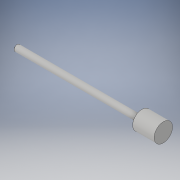
# Autodesk Inventor part: 5.4680.8730.50.500Double acting_00_005.4680.500.75N
Saved by Autodesk Inventor 2019 (Build 230136000, 136)
## iProperties
Created: 2023-02-15
Part Number: 5.4680.8730.50.500Double acting_00_005.4680.500.75N
Material: Generic
Catalog Web Link: www.cadenas.de
Description: SR Series Rod-Pneumatic Cylinder
Vendor: PARKERHANNIFIN
Document SubType Name: Modeling
Designer: psAdmin
Manufacturer: PARKERHANNIFIN
Mass: 10.4158 g
Surface Area: 44.7208 cm^2
Volume: 10.4158 cm^3
Density: 1 g/cm^3
Appearance: PSOLRGB-175-175-175
Category: PARTsolutions
Company: PARKERHANNIFIN
Title: 0.755.4680.8730.50Double acting
Author: Cadenas PARTsolutions
Comments: Pneumatic Cylinder
PSOL_IDENT_0: {$CADENAS_DATA/23d-libs/parkerpdn/actuators_cylinders/pneumatic_cylinders/sr_series/parts/sr_rod.prj
PSOL_IDENT_1: },412 {VTYP=3D},{NB=5.4680.8730.50.500Double acting_00_005.4680.500.75N},{LINA=0.755.4680.8730.50Dou
PSOL_IDENT_2: ble acting},{NN=SR Series Rod},{DATE=26.07.2021 05:25:39},{GEOMDATE=23.03.2020 14:58:48},{VERSION=},
PSOL_IDENT_3: {LINEID=40},{WBVAR=DR,RODLEN,PL,THDLEN,THDLENE2,CUT,HR,X2D,CT,RES,RET,RETT,RETS,REA,REEL,RWF,RESE2,R
PSOL_IDENT_4: ETE2,RETTE2,REAE2,REELE2,RWFE2,RETSE2,RL,W,MNT},{WBNUMERIC=RODLEN,PL,THDLEN,THDLENE2,X2D,REA,REEL,RE
PSOL_IDENT_5: AE2,REELE2,RL,W}  {NB=5.4680.8730.50.500Double acting_00_005.4680.500.75N},{LINA=0.755.4680.8730.50D
PSOL_IDENT_6: ouble acting},{KT=DUMMY},{PN=0.755.4680.8730.50Double acting},{BORE=0.7500},{BORECON=0.7500},{DR=},{
PSOL_IDENT_7: KK=1/4-28 UNF},{NDM=0.2500},{TAB=UNF},{RODLEN=5.46800},{PL=0.87300},{PLMAX=5.26800},{THDLEN=0.50000}
PSOL_IDENT_8: ,{THDLENE2=0.50000},{CUT=},{CUTALG= '' , 'Without Cut' , 'W' , 'Wrench Flats' , 'H' , 'Hex' },{D=0.2
PSOL_IDENT_9: 200},{DHEX=0.25000},{CC=0.2500},{WFLEN=0.00000},{WFALG=0},{WFMAX=4.59500},{HR=},{HRALG= '' , 'N/A' }
PSOL_IDENT_10: ,{AF=0.00000},{X2D=0},{CT=Double acting},{PREALG= <'_' , 'Standard Piston Rod End'> , '3' , '3 - Non
PSOL_IDENT_11: -Standard Piston Rod End' },{RES=_},{RET=},{RETALG='','N/A'},{RETT=},{RETTALG='','N/A'},{RETS=},{RET
PSOL_IDENT_12: SALG='','N/A'},{REA=0.000},{REEL=0.000},{RWF=},{RWFALG='','N/A','0','Omit Wrench Flats','2','Normal
PSOL_IDENT_13: - 2 Wrench Flats','4','4 Wrench Flats','6','6 Wrench Flats'},{RESE2=_},{RETE2=},{RETTE2=},{REAE2=0.0
PSOL_IDENT_14: 00},{REELE2=0.000},{RWFE2=},{RETSE2ALG='','N/A'},{RETSE2=},{SANDM=0.00000},{THDESC=N/A},{THE2DESC=N/
PSOL_IDENT_15: A},{SANDME2=0.00000},{SMNDM=0.000},{SMNDME2=0.000},{NDMALG=0.250},{RL=5.468},{PDIST=5.468},{KKD=-0.1
PSOL_IDENT_16: 25},{KKDE2=0.125},{WF=},{WFE2=},{W=0.500},{WN=0.440},{WP=0.440},{WNR=0.690},{WR=0.500},{WD=0.500},{W
PSOL_IDENT_17: BFD=0.500},{WBRN=0.690},{WBRD=0.690},{WA=0.340},{WAP=0.320},{WBRR=0.750},{WFLEN2=0.00000},{WFALG2=0}
PSOL_IDENT_18: ,{MNTALG= 'N' , 'N - Nose Mount, Spring Return' , 'NR' , 'NR - Nose Mount, Spring Return, Hex Rod (n
PSOL_IDENT_19: on-rotating)' , 'NRP' , 'NRP - Pivot and Nose Mount, Spring Return, Hex Rod (non-rotating)' , 'P' , '
PSOL_IDENT_20: P - Pivot Mount, Spring Return' , 'R' , 'R - Nose Mount, Spring Extended' , 'RP' , 'RP - Pivot and N
PSOL_IDENT_21: ose Mount, Spring Extend' , 'D' , 'D - Nose Mount, Double Acting'  , 'DX' , 'DX - Threaded Both End,
PSOL_IDENT_22: Double Acting' ,'DP' , 'DP - Pivot and Nose Mount, Double Acting, Pivot Pin' , 'DXP' , 'DXP - Pivot
PSOL_IDENT_23: and Nose Mount, Double Acting, No Pivot Pin' ,  'A' , 'A - Nose Mount, Spring Return, Head Adjustab
PSOL_IDENT_24: le Stroke' , 'RA' , 'RA - Nose Mount, Spring Extend, Cap Adjustable Stroke' , 'AP' , 'AP - Pivot Mou
PSOL_IDENT_25: nt, Spring Return, Head Adjustable Stroke' , 'AR' , 'AR - Air Reservoirs' , 'BRN' , 'BRN - Rear Bloc
PSOL_IDENT_26: k Mount, Single Acting, Spring Return' , 'BRR' , 'BRR - Rear Block Mount, Single Acting, Spring Exte
PSOL_IDENT_27: nd' , 'BFD' , 'BFD - Front Block Mount, Double Acting' , 'BRD' , 'BRD - Rear Block Mount, Double Act
PSOL_IDENT_28: ing' , 'BFN' , 'BFN - Front Block Mount, Single Acting, Spring Return' , 'BFR' , 'BFR - Front Block
PSOL_IDENT_29: Mount, Single Acting, Spring Extend' , 'TRN' , 'TRN - Rear Trunnion Mount, Single Acting, Spring Ret
PSOL_IDENT_30: urn' , 'TRR' , 'TRR - Rear Trunnion Mount, Single Acting, Spring Extend' , 'TFD' , 'TFD - Front Trun
PSOL_IDENT_31: nion Mount, Double Acting' , 'TRD' , 'TRD - Rear Trunnion Mount, Double Acting' , 'TFN' , 'TFN - Fro
PSOL_IDENT_32: nt Trunnion Mount, Single Acting, Spring Return' , 'TFR' , 'TFR - Front Trunnion Mount, Single Actin
PSOL_IDENT_33: g, Spring Extend' },{MNT=N},{C=0.000},{C1=0.100},{REAALG=[0]},{REA2ALG=[0]},{REELALG=[0]},{REEL2ALG=
PSOL_IDENT_34: [0]},{RETE2ALG='','N/A'},{RETTE2ALG='','N/A'},{RFW= },{RFWE2= }
NB: 5.4680.8730.50.500Double acting_00_005.4680.500.75N
NN: SR Series Rod
NT: Pneumatic Cylinder
NBSYN: $DR.$RODLEN.$PL.$THDLEN.$THDLENE2.$CUT.$WFLEN.$HR.$X2D.$CT.$RES.$RET.$RETT.$RETS.$REA.$REEL.$RWF.$RESE2.$RETE2.$RETTE2.$REAE2.$REELE2.$RWFE2.$RETSE2.$RL.$W.$WFLEN2.$BORE.$MNT.
LINA: 0.755.4680.8730.50Double acting
CATALOG: Parker Pneumatic Division
BORE: 0.75
BORECON: 0.7500
DR: Without
KK: 1/4-28 UNF
NDM: 0.25
TAB: UNF
RODLEN: 5.468
PL: 0.873
THDLEN: 0.5
THDLENE2: 0.5
CUT: Without Cut
D: 0.22
DHEX: 0.25
CC: 0.25
WFLEN: 0
HR: N/A
AF: 0
X2D: 0
CT: Double acting
RES: Standard Piston Rod End
RET: N/A
RETT: N/A
RETS: N/A
REA: 0
REEL: 0
RWF: N/A
RESE2: Standard Piston Rod End
RETE2: N/A
RETTE2: N/A
REAE2: 0
REELE2: 0
RWFE2: N/A
RETSE2: N/A
SANDM: 0
SANDME2: 0
SMNDM: 0
SMNDME2: 0
RL: 5.468
PDIST: 5.468
W: 0.5
WN: 0.44
WP: 0.44
WNR: 0.69
WR: 0.5
WD: 0.5
WBFD: 0.5
WBRN: 0.69
WBRD: 0.69
WA: 0.34
WAP: 0.32
WBRR: 0.75
MNT: N - Nose Mount, Spring Return
C1: 0.1
SUPPLIER: PARKERHANNIFIN
ARTICLENO: 5.4680.8730.50.500Double acting_00_005.4680.500.75N
BOMINFO: 0.755.4680.8730.50Double acting
CREATOR: CADENAS GmbH
Autodesk Inventor part; units mm, degrees
sketch "Sketch_1" plane through (0, 0, 0) normal (0, 0, 1) x (1, 0, 0)
  line L0 (138.8872, 0) -> (0, 0)
  line L1 (0, 0) -> (0, 3.175)
  line L2 (0, 3.175) -> (138.8872, 3.175)
  line L3 (138.8872, 3.175) -> (138.8872, 0)
  line L4 (138.8872, 0) -> (0, 0)
  constraints: 10 end point
revolve "Revolution1" add sketch "Sketch_1" angle 360 about axis through (138.8872, 0, 0) along (1, 0, 0)
sketch "Sketch_3" plane through (0, 0, 0) normal (0, 0, 1) x (1, 0, 0)
  line L0 (138.8872, 0) -> (116.713, 0)
  line L1 (116.713, 0) -> (116.713, 9.525)
  line L2 (116.713, 9.525) -> (138.8872, 9.525)
  line L3 (138.8872, 9.525) -> (138.8872, 0)
  line L4 (138.8872, 0) -> (116.713, 0)
  constraints: 10 end point
revolve "Revolution2" add sketch "Sketch_3" angle 360 about axis through (138.8872, 0, 0) along (1, 0, 0)
sketch "Sketch_4" plane through (0, 0, 0) normal (0, 0, 1) x (1, 0, 0)
  line L0 (0, 0) -> (-12.7, 0)
  line L1 (-12.7, 0) -> (-12.7, 2.634)
  line L2 (-12.7, 2.634) -> (-12.159, 3.175)
  line L3 (-12.159, 3.175) -> (0, 3.175)
  line L4 (0, 3.175) -> (0, 0)
  line L5 (0, 0) -> (-12.7, 0)
  constraints: 12 end point
revolve "Revolution3" add sketch "Sketch_4" angle 360 about axis through (0, 0, 0) along (1, 0, 0)
ref_plane "a_XY" through (-12.7, 0, 0) normal (1, 0, 0) x (0, 0, -1)
ref_plane "a_YZ" through (-12.7, 0, 0) normal (0, 0, -1) x (0, 1, 0)
ref_plane "a_ZX" through (-12.7, 0, 0) normal (0, 1, 0) x (1, 0, 0)
ref_plane "c1_XY" through (0, 0, 0) normal (1, 0, 0) x (0, 0, -1)
ref_plane "c1_YZ" through (0, 0, 0) normal (0, 0, -1) x (0, 1, 0)
ref_plane "c1_ZX" through (0, 0, 0) normal (0, 1, 0) x (1, 0, 0)
ref_plane "cc1_XY" through (0, 0, -3.175) normal (1, 0, 0) x (0, 0, -1)
ref_plane "cc1_YZ" through (0, 0, -3.175) normal (0, 0, -1) x (0, 1, 0)
ref_plane "cc1_ZX" through (0, 0, -3.175) normal (0, 1, 0) x (1, 0, 0)
ref_plane "cc2_XY" through (0, 0, 3.175) normal (1, 0, 0) x (0, 0, -1)
ref_plane "cc2_YZ" through (0, 0, 3.175) normal (0, 0, -1) x (0, 1, 0)
ref_plane "cc2_ZX" through (0, 0, 3.175) normal (0, 1, 0) x (1, 0, 0)
ref_plane "kk_XY" through (-6.35, 0, 3.175) normal (1, 0, 0) x (0, 0, -1)
ref_plane "kk_YZ" through (-6.35, 0, 3.175) normal (0, 0, -1) x (0, 1, 0)
ref_plane "kk_ZX" through (-6.35, 0, 3.175) normal (0, 1, 0) x (1, 0, 0)
ref_plane "rod_XY" through (138.8872, 0, 0) normal (1, 0, 0) x (0, 0, -1)
ref_plane "rod_YZ" through (138.8872, 0, 0) normal (0, 0, -1) x (0, 1, 0)
ref_plane "rod_ZX" through (138.8872, 0, 0) normal (0, 1, 0) x (1, 0, 0)
body "Solid1"
